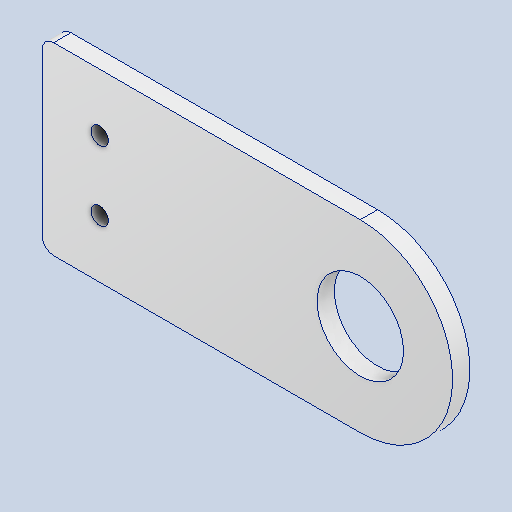
# Autodesk Inventor part: RZvector-v1-Plate-MM7-P-F-3
Saved by Autodesk Inventor 2025.1 (Build 291241000, 241)
## iProperties
Created: 2024-03-10
Part Number: RZvector-v1-Plate-MM7-P-F-3
Material: アルミニウム 6061
Document SubType Name: Modeling
Designer: haruy
Density: 2.7 g/cm^3
Appearance: アルミニウム - フラット
Author: haruy
Autodesk Inventor part; units mm, degrees
ref_plane "YZ Plane" through (0, 0, 0) normal (1, 0, 0) x (0, 1, 0)
ref_plane "XZ Plane" through (0, 0, 0) normal (0, 1, 0) x (-1, 0, 0)
ref_plane "XY Plane" through (0, 0, 0) normal (0, 0, 1) x (1, 0, 0)
derived "RZvector-v1-Sketch-Base.ipt"
sketch "横から" plane through (0, 0, 0) normal (0, 0, 1) x (1, 0, 0)
  line L0 (-165, 0) -> (-145, 0)
  line L1 (-145, 0) -> (-145, 594)
  line L2 (-145, 594) -> (-165, 594)
  line L3 (-165, 594) -> (-165, 0)
  line L4 (145, 0) -> (165, 0)
  line L5 (165, 0) -> (165, 594)
  line L6 (165, 594) -> (145, 594)
  line L7 (145, 594) -> (145, 0)
  circle A0 centre (200.18, 578) radius 16
  circle A1 centre (-200.18, 578) radius 16
  circle A2 centre (-200.18, 50) radius 16
  circle A3 centre (200.18, 50) radius 16
  circle A4 centre (-200.18, 82) radius 16
  line L8 (176.5, 164) -> (186.5, 164)
  line L9 (186.5, 164) -> (186.5, 134)
  line L10 (186.5, 134) -> (176.5, 134)
  line L11 (176.5, 134) -> (176.5, 164)
  circle A5 centre (200.18, 50) radius 13.68
  circle A6 centre (200.18, 578) radius 13.68
  line L12 (186.5, 50) -> (186.5, 578)
  line L13 (145, 0) -> (125, 0)
  line L14 (125, 0) -> (125, 20)
  line L15 (125, 20) -> (145, 20)
  line L16 (145, 20) -> (145, 0)
  line L17 (-230.4566, -34) -> (384.0946, -34)
  line L18 (125, 0) -> (165, 0)
  line L19 (165, 0) -> (165, -10)
  line L20 (165, -10) -> (125, -10)
  line L21 (125, -10) -> (125, 0)
  line L22 (176.5, 98) -> (-171.4306, 98)
  line L23 (-171.4306, 98) -> (-171.4306, 113)
  line L24 (-171.4306, 113) -> (176.5, 113)
  line L25 (176.5, 113) -> (176.5, 98)
  circle A7 centre (-200.18, 82) radius 13.68
  circle A8 centre (-200.18, 578) radius 13.68
  line L26 (-186.5, 164) -> (-176.5, 164)
  line L27 (-176.5, 164) -> (-176.5, 134)
  line L28 (-176.5, 134) -> (-186.5, 134)
  line L29 (-186.5, 134) -> (-186.5, 164)
  line L30 (-186.5, 578) -> (-186.5, 82)
  line L31 (-10, 142) -> (10, 142)
  line L32 (10, 142) -> (10, 122)
  line L33 (10, 122) -> (-10, 122)
  line L34 (-10, 122) -> (-10, 142)
  line L35 (-10, 526) -> (10, 526)
  line L36 (10, 526) -> (10, 506)
  line L37 (10, 506) -> (-10, 506)
  line L38 (-10, 506) -> (-10, 526)
  line L39 (-186.5, 539) -> (-176.5, 539)
  line L40 (-176.5, 539) -> (-176.5, 509)
  line L41 (-176.5, 509) -> (-186.5, 509)
  line L42 (-186.5, 509) -> (-186.5, 539)
  circle A9 centre (-232.18, 82) radius 16
  line L43 (-165, 0) -> (-145, 0)
  line L44 (-145, 0) -> (-145, -10)
  line L45 (-145, -10) -> (-165, -10)
  line L46 (-165, -10) -> (-165, 0)
  line L47 (145, 0) -> (145, -10)
  circle A10 centre (155, 44) radius 1.5
  circle A11 centre (155, 56) radius 1.5
  circle A12 centre (200.18, 50) radius 7.5
  line L48 (-145, 0) -> (-125, 0)
  line L49 (-125, 0) -> (-125, 20)
  line L50 (-125, 20) -> (-145, 20)
  line L51 (-145, 20) -> (-145, 0)
  line L52 (-200.18, 50) -> (-200.18, 34)
  circle A13 centre (-200.18, 50) radius 13.68
  line L53 (-200.18, 36.32) -> (200.18, 36.32)
  line L54 (200.18, 66) -> (145, 66)
  line L55 (200.18, 34) -> (145, 34)
  line L56 (145, 594) -> (165, 594)
  line L57 (165, 594) -> (165, 625.5)
  line L58 (165, 625.5) -> (145, 625.5)
  line L59 (145, 625.5) -> (145, 594)
  line L60 (-165, 594) -> (-145, 594)
  line L61 (-145, 594) -> (-145, 625.5)
  line L62 (-145, 625.5) -> (-165, 625.5)
  line L63 (-165, 625.5) -> (-165, 594)
  line L64 (200.18, 66) -> (145, 66)
  line L65 (200.18, 34) -> (145, 34)
  line L66 (130, 95.9) -> (157.8, 95.9)
  line L67 (157.8, 95.9) -> (157.8, 80)
  line L68 (157.8, 80) -> (130, 80)
  line L69 (130, 80) -> (130, 95.9)
  circle A14 centre (132.8, 93.1) radius 1.7
  circle A15 centre (155, 82.8) radius 1.7
  circle A16 centre (155, 74.8) radius 1.7
  line L70 (157.8, 95.9) -> (165, 95.9)
  line L71 (145, 69.8) -> (165, 69.8)
  line L72 (186.5, 539) -> (176.5, 539)
  line L73 (176.5, 539) -> (176.5, 509)
  line L74 (176.5, 509) -> (186.5, 509)
  line L75 (186.5, 509) -> (186.5, 539)
  line L76 (152.2, 557) -> (180, 557)
  line L77 (180, 557) -> (180, 541.1)
  line L78 (180, 541.1) -> (152.2, 541.1)
  line L79 (152.2, 541.1) -> (152.2, 557)
  line L80 (175.1, 557) -> (175.1, 541.1)
  circle A17 centre (155, 543.9) radius 1.7
  circle A18 centre (177.2, 554.2) radius 1.7
  circle A19 centre (155, 535.9) radius 1.7
  line L81 (152.2, 557) -> (145, 557)
  line L82 (145, 530.9) -> (165, 530.9)
  point P0 (0, 0)
  point P1 (165, 20)
  point P2 (145, 40)
  point P3 (165, 40)
  point P4 (202.3646, 34.1498)
  point P5 (192.5041, 64.0385)
  dimension "d1" = 3
  dimension "d2" = 3
  dimension "d3" = 15
  dimension "d7" = 10
  dimension "d8" = 10
  dimension "d11" = 10
  dimension "d12" = 10
  measures "d1" diameter of A10
  measures "d2" diameter of A11
  measures "d3" diameter of A12
  measures "d7" distance from line of A11.centre L5
  measures "d8" distance from line of A10.centre L5
  measures "d11" distance from line of A11.centre L54
  measures "d12" distance from line of A10.centre L55
sketch "上から" plane through (0, 0, 0) normal (0, 1, 0) x (-1, 0, 0)
  line L0 (0, 0) -> (20, 0)
  line L1 (20, 0) -> (20, -20)
  line L2 (20, -20) -> (0, -20)
  line L3 (0, -20) -> (0, 0)
  line L4 (0, -220) -> (20, -220)
  line L5 (20, -220) -> (20, -240)
  line L6 (20, -240) -> (0, -240)
  line L7 (0, -240) -> (0, -220)
  line L8 (16.25, -259.18) -> (3.75, -259.18)
  line L9 (3.75, -259.18) -> (3.75, -291.18)
  line L10 (3.75, -291.18) -> (16.25, -291.18)
  line L11 (16.25, -291.18) -> (16.25, -259.18)
  line L12 (16.25, 19.18) -> (3.75, 19.18)
  line L13 (3.75, 19.18) -> (3.75, 51.18)
  line L14 (3.75, 51.18) -> (16.25, 51.18)
  line L15 (16.25, 51.18) -> (16.25, 19.18)
  line L16 (20, -220) -> (22, -220)
  line L17 (22, -220) -> (22, -358.5675)
  line L18 (22, -358.5675) -> (20, -358.5675)
  line L19 (20, -358.5675) -> (20, -220)
  line L20 (0, -220) -> (-2, -220)
  line L21 (-2, -220) -> (-2, -291.18)
  line L22 (-2, -291.18) -> (0, -291.18)
  line L23 (0, -291.18) -> (0, -220)
  line L24 (-7, -282.2193) -> (-7, -294.2193)
  line L25 (-7, -259.18) -> (-19.5, -259.18)
  line L26 (-19.5, -259.18) -> (-19.5, -291.18)
  line L27 (-19.5, -291.18) -> (-7, -291.18)
  line L28 (-7, -291.18) -> (-7, -259.18)
  line L29 (20, -20) -> (22, -20)
  line L30 (22, -20) -> (22, 104.8767)
  line L31 (22, 104.8767) -> (20, 104.8767)
  line L32 (20, 104.8767) -> (20, -20)
  line L33 (0, -20) -> (-2, -20)
  line L34 (-2, -20) -> (-2, 45.2504)
  line L35 (-2, 45.2504) -> (0, 45.2504)
  line L36 (0, 45.2504) -> (0, -20)
  line L37 (45, 41.18) -> (-19.5, 41.18)
  line L38 (-19.5, 41.18) -> (-19.5, 29.18)
  line L39 (-19.5, 29.18) -> (45, 29.18)
  line L40 (45, 29.18) -> (45, 41.18)
  line L41 (16.25, -275.18) -> (3.75, -275.18)
  line L42 (16.25, 35.18) -> (3.75, 35.18)
  line L43 (20, -20) -> (22, -20)
  line L44 (22, -20) -> (22, -20)
  line L45 (22, -20) -> (20, -20)
  line L46 (20, -20) -> (20, -20)
  line L47 (0, -20) -> (-2, -20)
  line L48 (-2, -20) -> (-2, -20)
  line L49 (-2, -20) -> (0, -20)
  line L50 (0, -20) -> (0, -20)
  line L51 (20, 79.43) -> (-14.5, 79.43)
  line L52 (-14.5, 79.43) -> (-14.5, 54.93)
  line L53 (-14.5, 54.93) -> (20, 54.93)
  line L54 (20, 54.93) -> (20, 79.43)
  line L55 (20, 73.18) -> (22, 73.18)
  line L56 (22, 73.18) -> (22, 61.18)
  line L57 (22, 61.18) -> (20, 61.18)
  line L58 (20, 61.18) -> (20, 73.18)
  line L59 (22, 69.18) -> (32, 69.18)
  line L60 (32, 69.18) -> (32, 65.18)
  line L61 (32, 65.18) -> (22, 65.18)
  line L62 (22, 65.18) -> (22, 69.18)
  line L63 (-14.5, 67.18) -> (20, 67.18)
  line L64 (-7, 51.18) -> (-19.5, 51.18)
  line L65 (-19.5, 51.18) -> (-19.5, 19.18)
  line L66 (-19.5, 19.18) -> (-7, 19.18)
  line L67 (-7, 19.18) -> (-7, 51.18)
  line L68 (35, 47.68) -> (29, 47.68)
  line L69 (29, 47.68) -> (29, 22.68)
  line L70 (29, 22.68) -> (35, 22.68)
  line L71 (35, 22.68) -> (35, 47.68)
  line L72 (45, 51.18) -> (35, 51.18)
  line L73 (35, 51.18) -> (35, 19.18)
  line L74 (35, 19.18) -> (45, 19.18)
  line L75 (45, 19.18) -> (45, 51.18)
  line L76 (45, 83.18) -> (35, 83.18)
  line L77 (35, 83.18) -> (35, 51.18)
  line L78 (35, 51.18) -> (45, 51.18)
  line L79 (45, 51.18) -> (45, 83.18)
  line L80 (-7, -275.18) -> (-19.5, -275.18)
  line L81 (42, -269.18) -> (-19.5, -269.18)
  line L82 (-19.5, -269.18) -> (-19.5, -281.18)
  line L83 (-19.5, -281.18) -> (42, -281.18)
  line L84 (42, -281.18) -> (42, -269.18)
  line L85 (20, -301.68) -> (-79, -301.68)
  line L86 (-79, -301.68) -> (-79, -348.68)
  line L87 (-79, -348.68) -> (20, -348.68)
  line L88 (20, -348.68) -> (20, -301.68)
  line L89 (20, -312.68) -> (22, -312.68)
  line L90 (22, -312.68) -> (22, -337.68)
  line L91 (22, -337.68) -> (20, -337.68)
  line L92 (20, -337.68) -> (20, -312.68)
  line L93 (22, -321.18) -> (42, -321.18)
  line L94 (42, -321.18) -> (42, -329.18)
  line L95 (42, -329.18) -> (22, -329.18)
  line L96 (22, -329.18) -> (22, -321.18)
  line L97 (42, -259.18) -> (32, -259.18)
  line L98 (32, -259.18) -> (32, -291.18)
  line L99 (32, -291.18) -> (42, -291.18)
  line L100 (42, -291.18) -> (42, -259.18)
  line L101 (42, -309.18) -> (32, -309.18)
  line L102 (32, -309.18) -> (32, -341.18)
  line L103 (32, -341.18) -> (42, -341.18)
  line L104 (42, -341.18) -> (42, -309.18)
  line L105 (22, -325.18) -> (42, -325.18)
  line L106 (32, -262.68) -> (26, -262.68)
  line L107 (26, -262.68) -> (26, -287.68)
  line L108 (26, -287.68) -> (32, -287.68)
  line L109 (32, -287.68) -> (32, -262.68)
  point P0 (10, 35.18)
extrude "押し出し1" add sketch "横から" along normal blind 3 contours L53 L5 L55 L7 | L7 L54 L5 L53 | L53 A3 L55 L5 | L5 L54 L12 A3 L53 | L53 A5 L12 A3 | A3 L12 A5 L53 | L54 A3 L12 | A5
fillet "フィレット1" radius 2 2 edges at (145, 66, 1.5) (145, 34, 1.5)
sketch "スケッチ3" plane through (200.18, 50, 3) normal (0, 0, 1) x (1, 0, 0)
  arc A0 (-55.18, -14) -> (-53.18, -16) centre (-53.18, -14) ccw projected
  line L0 (-53.18, -16) -> (0, -16) projected
  arc A1 (0, -16) -> (0, 16) centre (0, 0) ccw projected
  line L1 (0, 16) -> (-53.18, 16) projected
  arc A2 (-53.18, 16) -> (-55.18, 14) centre (-53.18, 14) ccw projected
  line L2 (-55.18, 14) -> (-55.18, -14) projected
  circle A3 centre (0, 0) radius 7.5 projected
  circle A4 centre (-45.18, -6) radius 1.5 projected
  circle A5 centre (-45.18, 6) radius 1.5 projected
  point P0 (-200.18, -50)
